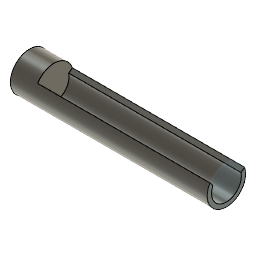
cat-dispenser-center-fusion (Autodesk Fusion 360 design; units mm, degrees)
Autodesk Fusion 360 part; units mm, degrees
sketch "Esboço1" plane through (0, 0, 0) normal (1, 0, 0) x (0, 1, 0)
  circle A0 centre (0, 0) radius 11.75
  dimension "d1" = 23.5
  constraint coincident A0.centre origin
  measures "d1" diameter of A0
extrude "Extrusão1" add sketch "Esboço1" along normal blind 120
sketch "Esboço2" plane through (120, 0, 0) normal (1, 0, 0) x (0, 1, 0)
  circle A0 centre (0, 0) radius 11.75
sketch "Esboço3" plane through (120, 0, 0) normal (1, 0, 0) x (0, 1, 0)
  line L0 (-10, 6) -> (-8.3006, 3.7257)
  line L1 (11.1508, 3.7257) -> (8.8709, 2.0221)
  arc A0 (-8.3006, 3.7257) -> (8.8709, 2.0221) centre (0, 0) ccw
  line L2 (-10.8021, 6.8786) -> (-10, 6)
  line L3 (11.8471, 4.8629) -> (11.1508, 3.7257)
  arc A1 (11.8471, 4.8629) -> (-10.8021, 6.8786) centre (0, 0) ccw
  arc A2 (-10.062, 6.0679) -> (11.1451, 3.7214) centre (0, 0) ccw
  dimension "d4" = 23.5
  constraint coincident A0.centre A1.centre
  constraint perpendicular L0 L1
  constraint concentric A0 A2
  constraint concentric A1 A2
  constraint coincident L1 A2.end
  constraint coincident L2 A2.start
  measures "d4" diameter of A2
extrude "Extrusão2" cut sketch "Esboço3" against normal blind 105 contours L0 L1 A0 L2 L3 A1
